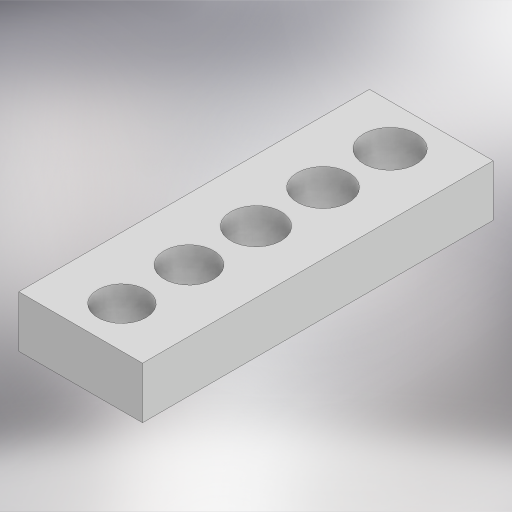
# Autodesk Inventor part: Testbed
Saved by Autodesk Inventor 2024.3 (Build 283343000, 343)
## iProperties
Created: 2025-04-26
Part Number: Testbed
Material: Generic
Document SubType Name: Modeling
Designer: danie
Density: 1 g/cm^3
Appearance: Default
Author: danie
Autodesk Inventor part; units mm, degrees
ref_plane "YZ Plane" through (0, 0, 0) normal (1, 0, 0) x (0, 1, 0)
ref_plane "XZ Plane" through (0, 0, 0) normal (0, 1, 0) x (-1, 0, 0)
ref_plane "XY Plane" through (0, 0, 0) normal (0, 0, 1) x (1, 0, 0)
sketch "Sketch1" plane through (0, 0, 0) normal (0, 1, 0) x (-1, 0, 0)
  line L0 (-6, 17) -> (6, 17)
  line L1 (6, 17) -> (6, -17)
  line L2 (6, -17) -> (-6, -17)
  line L3 (-6, -17) -> (-6, 17)
  line L4 (-6, 17) -> (6, -17) construction
  line L5 (6, 17) -> (-6, -17) construction
  line L6 (0, 17) -> (0, -17)
  circle A0 centre (0, -13) radius 2.55
  circle A1 centre (0, -6.5) radius 2.5
  circle A2 centre (0, 0) radius 2.45
  circle A3 centre (0, 6.5) radius 2.4
  circle A4 centre (0, 13) radius 2.35
  point P0 (0, 0)
  dimension "d0" = 12
  dimension "d1" = 34
  dimension "d2" = 4
  dimension "d3" = 5.1
  dimension "d4" = 6.5
  dimension "d5" = 5
  dimension "d6" = 6.5
  dimension "d7" = 4.9
  dimension "d8" = 6.5
  dimension "d9" = 4.8
  dimension "d10" = 6.5
  dimension "d11" = 4.7
  constraints: 14 end point, 5 centre point, 5 midpoint, 4 point on line, 2 parallel, 1 horizontal, 1 perpendicular
  measures "d0" distance between parallel lines of L3 L1
  measures "d1" distance between parallel lines of L2 L0
  measures "d2" distance from line of L2 A0.centre
  measures "d3" diameter of A0
  measures "d4" distance of A1.centre A0.centre
  measures "d5" diameter of A1
  measures "d6" distance of A2.centre A1.centre
  measures "d7" diameter of A2
  measures "d8" distance of A2.centre A3.centre
  measures "d9" diameter of A3
  measures "d10" distance of A3.centre A4.centre
  measures "d11" diameter of A4
extrude "Extrusion1" add sketch "Sketch1" along normal blind 5 contours L0 L6 A4 A3 A2 A1 A0 L2 L3 | L0 L1 L2 L6 A0 A1 A2 A3 A4
body "Solid1"
